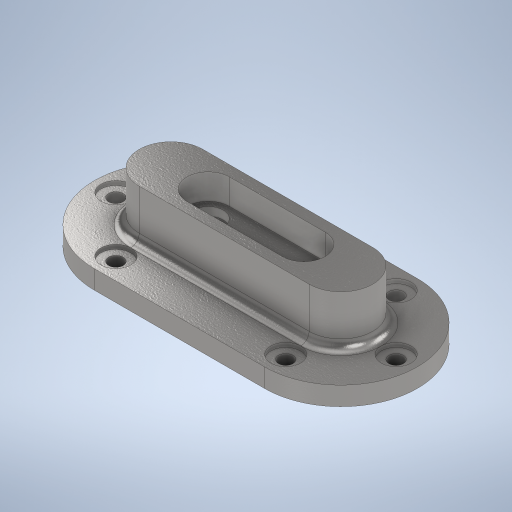
# Autodesk Inventor part: Bauteil2
Saved by Autodesk Inventor 2024 (Build 280153000, 153)
## iProperties
Created: 2024-02-02
Part Number: Bauteil2
Material: Stahl, galvanisiert
Document SubType Name: Modeling
Designer: ffogue
Density: 7.85 g/cm^3
Appearance: Galvanisiert
Author: ffogue
Autodesk Inventor part; units mm, degrees
ref_plane "YZ Plane" through (0, 0, 0) normal (1, 0, 0) x (0, 1, 0)
ref_plane "XZ Plane" through (0, 0, 0) normal (0, 1, 0) x (-1, 0, 0)
ref_plane "XY Plane" through (0, 0, 0) normal (0, 0, 1) x (1, 0, 0)
sketch "Skizze1" plane through (0, 0, 0) normal (0, 0, 1) x (1, 0, 0)
  line L0 (-20, 36) -> (20, 36)
  line L1 (38, 18) -> (38, 18)
  line L2 (20, 0) -> (-20, 0)
  line L3 (-38, 18) -> (-38, 18)
  arc A0 (-20, 36) -> (-38, 18) centre (-20, 18) ccw
  arc A1 (-38, 18) -> (-20, 0) centre (-20, 18) ccw
  arc A2 (38, 18) -> (20, 36) centre (20, 18) ccw
  arc A3 (20, 0) -> (38, 18) centre (20, 18) ccw
  point P0 (0, 0)
  point P1 (0, 0)
  point P2 (38, 18)
  dimension "d0" = 36
  dimension "d1" = 18
  dimension "d2" = 40
  constraints: 8 end point, 8 point on circle, 8 tangent, 4 centre point, 3 equal radius, 2 parallel, 1 coincident, 1 horizontal, 1 midpoint, 1 perpendicular
  measures "d0" distance between parallel lines of L2 L0
  measures "d1" radius of A0
  measures "d2" distance of A3.centre A0.centre
extrude "Extrusion1" add sketch "Skizze1" along normal blind 4.4
sketch "Skizze2" plane through (0, 0, 4.4) normal (0, 0, 1) x (1, 0, 0)
  line L0 (-11.25, 18) -> (11.25, 18) construction
  line L1 (-11.25, 23) -> (11.25, 23)
  line L2 (11.25, 13) -> (-11.25, 13)
  arc A0 (-11.25, 23) -> (-11.25, 13) centre (-11.25, 18) ccw
  arc A1 (11.25, 13) -> (11.25, 23) centre (11.25, 18) ccw
  arc A2 (-20, 36) -> (-20, 0) centre (-20, 18) ccw projected
  line L3 (-20, 0) -> (20, 0) projected
  line L4 (-20, 18) -> (20, 18) construction
  line L5 (-20, 10.5) -> (20, 10.5)
  line L6 (20, 25.5) -> (-20, 25.5)
  arc A3 (-20, 25.5) -> (-20, 10.5) centre (-20, 18) ccw
  arc A4 (20, 10.5) -> (20, 25.5) centre (20, 18) ccw
  point P0 (0, 0)
  point P1 (0, 18)
  point P2 (-38, 18)
  point P3 (0, 0)
  point P4 (0, 18)
  dimension "d5" = 22.5
  dimension "d6" = 5
  dimension "d7" = 7.5
  constraints: 16 end point, 9 point on circle, 8 tangent, 4 centre point, 3 midpoint, 2 parallel, 1 coincident, 1 horizontal, 1 horizontal alignment, 1 point on line, 1 vertical alignment
  measures "d5" distance of L0.end L0.start
  measures "d6" radius of A0
  measures "d7" radius of A3
extrude "Extrusion3" add sketch "Skizze2" along normal blind 5.6 contours L1 A1 L2 A0
extrude "Extrusion4" add sketch "Skizze2" along normal blind 11.6
fillet "Rundung1" radius 2 4 edges at (27.5, 18, 4.4) (0, 10.5, 4.4) (-27.5, 18, 4.4) (0, 25.5, 4.4)
sketch "Skizze3" plane through (0, 0, 10) normal (0, 0, 1) x (1, 0, 0)
  arc A0 (-11.25, 23) -> (-11.25, 13) centre (-11.25, 18) ccw projected
  point P0 (0, 0)
  constraints: 1 coincident
hole "Bohrung1" at (-11.25, 18, 10) direction (0, 0, -1) diameter 5 depth 10 counterbore diameter 7 counterbore depth 2
sketch "Skizze4" plane through (0, 0, 10) normal (0, 0, 1) x (1, 0, 0)
  arc A0 (11.25, 13) -> (11.25, 23) centre (11.25, 18) ccw projected
  point P0 (0, 0)
  constraints: 1 coincident
hole "Bohrung2" at (11.25, 18, 10) direction (0, 0, -1) diameter 5 depth 10 counterbore diameter 7 counterbore depth 2
sketch "Skizze5" plane through (0, 0, 4.4) normal (0, 0, 1) x (1, 0, 0)
  arc A0 (-20, 31) -> (-20, 5) centre (-20, 18) ccw construction
  line L0 (-20, 31) -> (20, 31) construction
  arc A1 (20, 10.5) -> (20, 25.5) centre (20, 18) ccw construction
  line L1 (20, 25.5) -> (-20, 25.5) construction
  arc A2 (-20, 25.5) -> (-20, 10.5) centre (-20, 18) ccw construction
  line L2 (-20, 10.5) -> (20, 10.5) construction
  line L3 (11.25, 13) -> (-11.25, 13) construction
  arc A3 (-11.25, 23) -> (-11.25, 13) centre (-11.25, 18) ccw construction
  line L4 (-11.25, 23) -> (11.25, 23) construction
  arc A4 (11.25, 13) -> (11.25, 23) centre (11.25, 18) ccw construction
  arc A5 (20, 5) -> (20, 31) centre (20, 18) ccw construction
  line L5 (-20, 5) -> (20, 5) construction
  arc A6 (-20, 27.5) -> (-20, 8.5) centre (-20, 18) ccw construction
  point P0 (0, 0)
  point P1 (20, 8.5)
  point P2 (-33, 18)
  point P3 (33, 18)
  dimension "d30" = 13
  constraints: 6 point on circle, 4 coincident, 4 end point, 2 centre point, 2 horizontal, 2 vertical alignment, 1 concentric, 1 equal radius, 1 parallel, 1 tangent
  measures "d30" radius of A0
hole "Bohrung3" at (-33, 18, 4.4) at (33, 18, 4.4) at (-20, 31, 4.4) at (-20, 5, 4.4) at (20, 31, 4.4) at (20, 5, 4.4) direction (0, 0, -1) diameter 3.4 end through all counterbore diameter 7 counterbore depth 1
